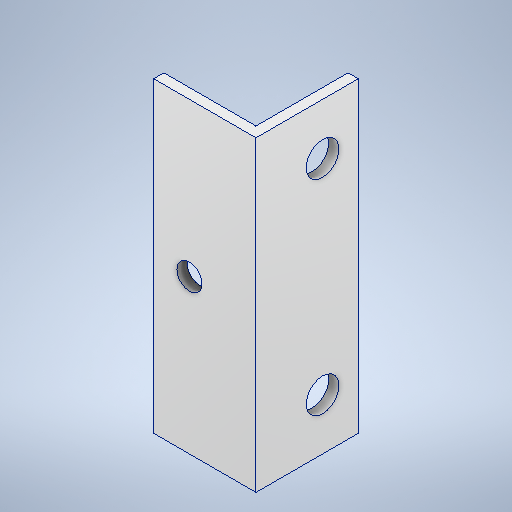
# Autodesk Inventor part: y_cable_adaptor_holder
Saved by Autodesk Inventor 2025 (Build 290162000, 162)
## iProperties
Created: 2024-04-25
Part Number: y_cable_adaptor_holder
Material: Hliník 6061
Document SubType Name: Modeling
Designer: rader
Density: 2.7 g/cm^3
Appearance: Hliník – plochý
Author: rader
Autodesk Inventor part; units mm, degrees
ref_plane "YZ Plane" through (0, 0, 0) normal (1, 0, 0) x (0, 1, 0)
ref_plane "XZ Plane" through (0, 0, 0) normal (0, 1, 0) x (-1, 0, 0)
ref_plane "XY Plane" through (0, 0, 0) normal (0, 0, 1) x (1, 0, 0)
sketch "Náčrt1" plane through (0, 0, 0) normal (0, 0, 1) x (1, 0, 0)
  line L0 (-10, 0) -> (0, 0)
  line L1 (0, 0) -> (0, 10)
  line L2 (0, 10) -> (-1, 10)
  line L3 (-1, 10) -> (-1, 1)
  line L4 (-1, 1) -> (-10, 1)
  line L5 (-10, 1) -> (-10, 0)
  line L6 (0, 12) -> (0, -2) projected
  line L7 (-12, 0) -> (2, 0) projected
  point P0 (0, 0)
  dimension "d0" = 10
  dimension "d1" = 10
  dimension "d2" = 1
  dimension "d3" = 1
  constraints: 12 end point, 5 perpendicular, 2 collinear, 1 horizontal
  measures "d0" distance of L0.start L0.end
  measures "d1" distance of L0.end L1.end
  measures "d2" distance between parallel lines of L3 L1
  measures "d3" distance between parallel lines of L4 L0
extrude "Vysunutí1" add sketch "Náčrt1" along normal mid plane 30
sketch "Náčrt2" plane through (0, 0, 15) normal (1, 0, 0) x (0, 0, -1)
  line L0 (30, 10) -> (0, 10) projected
  line L1 (30, 10) -> (30, 0) projected
  point P0 (15, 0)
  point P1 (5, 6.5)
  point P2 (25, 6.5)
  point P3 (30, 5)
  dimension "d6" = 3.5
  dimension "d7" = 3.5
  dimension "d8" = 20
  dimension "d9" = 5
  constraints: 1 midpoint
  measures "d6" distance from line of L0 point (25, 6.5)
  measures "d7" distance from line of L0 point (5, 6.5)
  measures "d8" distance of point (25, 6.5) point (5, 6.5)
  measures "d9" horizontal distance of point (30, 5) point (25, 6.5)
hole "Díra1" at (0, 6.5, 10) at (0, 6.5, -10) direction (-1, 0, 0) diameter 3.2 end through all
sketch "Náčrt3" plane through (-10, 1, 15) normal (0, 1, 0) x (1, 0, 0)
  line L0 (0, 0) -> (0, 30) projected
  line L1 (0, 0) -> (0, 30) projected
  line L2 (9, 0) -> (0, 0) projected
  line L3 (9, 30) -> (9, 0) projected
  line L4 (0, 30) -> (9, 30) projected
  point P0 (10, 15)
  point P1 (3.5, 15)
  dimension "d17" = 3.5
  dimension "d18" = 15
  measures "d17" distance from line of L0 point (3.5, 15)
  measures "d18" distance from line of L2 point (3.5, 15)
hole "Díra2" at (-6.5, 1, 0) direction (0, -1, 0) diameter 2.459 end through all thread size "M3x0.5" class "6H" standard "ISO Metric profile"
